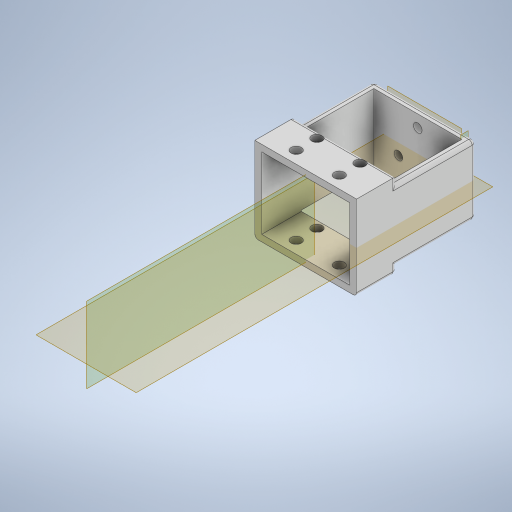
# Autodesk Inventor part: gripper-adapter
Saved by Autodesk Inventor 2024 (Build 280153000, 153)
## iProperties
Created: 2024-04-26
Part Number: gripper-adapter
Material: Generic
Document SubType Name: Modeling
Designer: MaartenGeorgesBuelen
Density: 1 g/cm^3
Appearance: Default
Author: MaartenGeorgesBuelen
## iProperties of the stored document gripper-adapter_3DPrint.ipt
Created: 2024-04-26
Part Number: gripper-adapter_3DPrint
Material: Generic
Document SubType Name: Modeling
Designer: MaartenGeorgesBuelen
Density: 1 g/cm^3
Appearance: Default
Author: MaartenGeorgesBuelen
Autodesk Inventor part; units mm, degrees
ref_plane "YZ Plane" through (0, 0, 0) normal (1, 0, 0) x (0, 1, 0)
ref_plane "XZ Plane" through (0, 0, 0) normal (0, 1, 0) x (-1, 0, 0)
ref_plane "Work Plane1" through (0, 0, 0) normal (0, 0, 1) x (1, 0, 0)
ref_plane "Work Plane7" through (25, -7, 170) normal (-1, 0, 0) x (0, 0, -1)
sketch "Sketch1" plane through (0, 0, 0) normal (0, 0, 1) x (1, 0, 0)
  circle A0 centre (0, 13) radius 5 projected
  line L0 (-15.25, 21.0877) -> (-12.5, 22.6754) projected
  line L1 (-12.5, 22.6754) -> (-9.75, 21.0877) projected
  line L2 (-9.75, 21.0877) -> (-9.75, 17.9123) projected
  line L3 (-9.75, 17.9123) -> (-12.5, 16.3246) projected
  line L4 (-12.5, 16.3246) -> (-15.25, 17.9123) projected
  line L5 (-15.25, 17.9123) -> (-15.25, 21.0877) projected
  line L6 (9.75, 21.0877) -> (12.5, 22.6754) projected
  line L7 (12.5, 22.6754) -> (15.25, 21.0877) projected
  line L8 (15.25, 21.0877) -> (15.25, 17.9123) projected
  line L9 (15.25, 17.9123) -> (12.5, 16.3246) projected
  line L10 (12.5, 16.3246) -> (9.75, 17.9123) projected
  line L11 (9.75, 17.9123) -> (9.75, 21.0877) projected
  circle A1 centre (-11.2583, 6.5) radius 1.5 projected
  circle A2 centre (11.2583, 6.5) radius 1.5 projected
  circle A3 centre (0, 26) radius 1.5 projected
  line L12 (-16.5, -4) -> (16.5, -4) projected
  line L13 (16.5, -4) -> (16.5, 0.0385) projected
  arc A4 (17.5169, 4.4322) -> (16.5, 0.0385) centre (26.5, 0.0385) ccw projected
  arc A5 (17.5169, 4.4322) -> (-17.5169, 4.4322) centre (0, 13) ccw projected
  arc A6 (-16.5, 0.0385) -> (-17.5169, 4.4322) centre (-26.5, 0.0385) ccw projected
  line L14 (-16.5, 0.0385) -> (-16.5, -4) projected
  line L15 (0, 39.8) -> (0, -11.3)
  line L16 (16.5, -7) -> (16.5, 33)
  line L17 (-5, -7) -> (-25, -7) projected
  line L18 (-25, 33) -> (-5, 33) projected
  line L19 (16.5, -7) -> (29.5, -7)
  line L20 (29.5, -7) -> (29.5, 33)
  line L21 (29.5, 33) -> (16.5, 33)
  line L22 (16.5, 33) -> (16.5, -7)
  line L23 (25, -21.52) -> (25, 50.02) projected
  line L24 (-16.5, -4) -> (-16.5, 0.0385)
  line L25 (-16.5, -7) -> (-16.5, 33)
  line L26 (-16.5, -7) -> (-29.5, -7)
  line L27 (-29.5, -7) -> (-29.5, 33)
  line L28 (-29.5, 33) -> (-16.5, 33)
  line L29 (-16.5, 33) -> (-16.5, -7)
  line L30 (16.5, -7) -> (-16.5, -7)
  line L31 (-16.5, 33) -> (16.7576, 33)
  circle A7 centre (11.2583, 6.5) radius 2.5
  circle A8 centre (-11.2583, 6.5) radius 2.5
  circle A9 centre (0, 26) radius 2.5
  point P0 (0, 0)
  point P1 (16.5, 23.3923)
  point P2 (-11.2583, 6.5)
  point P3 (-26.5, 0.0385)
  point P4 (25, -7)
  point P5 (25, 33)
  point P6 (-5, 33)
  dimension "d28" = 4.5
  dimension "d29" = 40
  dimension "d30" = 60
  dimension "d31" = 40
  dimension "d32" = 41.5
  dimension "d33" = 12.4413
  dimension "d34" = 8.5
  dimension "d35" = 4.1208
  dimension "d36" = 8.5
  dimension "d37" = 16.1041
  dimension "d38" = 8.5
  dimension "d39" = 16.1041
  dimension "d40" = 8.5
  dimension "d41" = 19.6016
  dimension "d60" = 1
  dimension "d61" = 1
  dimension "d62" = 1
  constraints: 28 end point, 7 symmetric about line, 3 centre point, 2 parallel, 1 collinear, 1 horizontal, 1 perpendicular, 1 point on line, 1 vertical, 2 other
  measures "d28" distance between parallel lines of L23 L20
  measures "d29" distance between parallel lines of L19 L21
  measures "d30" angle of L9 L25
  measures "d31" distance between parallel lines of L17 L21
  measures "d32" distance between parallel lines of L23 L29
  measures "d33" distance from line of L16.end L9
  measures "d34" distance from line of point (16.5, 23.392) L23
  measures "d35" distance from line of point (16.5, 23.392) L9
  measures "d36" distance from line of point (16.5, 0.039) L23
  measures "d37" distance from line of point (16.5, 0.039) L9
  measures "d38" distance from line of point (16.5, 0.039) L23
  measures "d39" distance from line of point (16.5, 0.039) L9
  measures "d40" distance from line of point (16.5, -4) L23
  measures "d41" distance from line of point (16.5, -4) L9
  measures "d60" radial gap between concentric circles of A2 A7
  measures "d61" radial gap between concentric circles of A1 A8
  measures "d62" radial gap between concentric circles of A3 A9
extrude "Extrusion1" add sketch "Sketch1" along normal blind 4 contours A0 L15 | A0 L15 A9 A5 L16 L13 L12 | L15 A0 | A0 L15 L12 L14 L25 A5 A9 | L15 L30 L17 L25 L12 | L12 L16 L30 L15 | L25 L17 L26 L27 L28 L18 A5 A6 L14 | L13 A4 A5 L16 L21 L23 L19 | L15 L31 L16 A5 | A5 L25 L18 L31 L15 | A6 A5 L25 | L16 A5 A4 | L23 L21 L20 L19 | L0 L1 L2 L3 L4 L5 | L6 L7 L8 L9 L10 L11
sketch "Sketch6" plane through (0, 0, 4) normal (0, 0, 1) x (1, 0, 0)
  line L0 (-29.5, 33) -> (-29.5, -7) projected
  line L1 (29.5, -7) -> (25.5, -7)
  line L2 (25.5, -7) -> (25.5, 33)
  line L3 (25.5, 33) -> (29.5, 33)
  line L4 (29.5, 33) -> (29.5, -7)
  line L5 (-29.5, -7) -> (-25.5, -7)
  line L6 (-25.5, -7) -> (-25.5, 33)
  line L7 (-25.5, 33) -> (-29.5, 33)
  line L8 (-29.5, 33) -> (-29.5, -7)
  line L9 (-29.5, -7) -> (29.5, -7) projected
  line L10 (29.5, -7) -> (29.5, 33) projected
  line L11 (29.5, 33) -> (-29.5, 33) projected
  point P0 (0, 0)
  dimension "d42" = 4
  dimension "d43" = 4
  dimension "d44" = 0
  dimension "d45" = 0
  constraints: 16 end point, 4 parallel, 2 horizontal, 2 perpendicular
  measures "d42" distance of L2.end L3.end
  measures "d43" distance of L7.end L6.end
  measures "d44" distance between parallel lines of L11 L3
  measures "d45" distance between parallel lines of L11 L7
extrude "Extrusion6" add sketch "Sketch6" along normal blind 65 contours L3 L4 L1 L2
sketch "Sketch7" plane through (-29.5, -7, 0) normal (0, -1, 0) x (1, 0, 0)
  line L0 (55, 69) -> (59, 69) projected
  line L1 (59, 0) -> (59, 69) projected
  line L2 (55, 69) -> (59, 69)
  line L3 (59, 69) -> (59, 46)
  line L4 (59, 46) -> (55, 46)
  line L5 (55, 46) -> (55, 69)
  point P0 (29.5, 0)
  dimension "d48" = 23
  constraints: 8 end point, 2 parallel, 1 horizontal, 1 perpendicular, 1 point on line
  measures "d48" distance of L2.end L3.end
extrude "Extrusion7" add sketch "Sketch7" along normal blind 4.5
sketch "Sketch8" plane through (25.5, -7, 4) normal (-1, 0, 0) x (0, 0, 1)
  line L0 (0, 0) -> (0, 40) projected
  line L1 (0, 0) -> (42, 0) projected
  line L2 (42, 0) -> (42, -4.5) projected
  line L3 (65, -4.5) -> (42, -4.5) projected
  line L4 (65, 40) -> (65, -4.5) projected
  line L5 (0, 40) -> (65, 40) projected
  line L6 (65, -4.5) -> (42, -4.5)
  line L7 (42, -4.5) -> (42, -0.7)
  line L8 (42, -0.7) -> (65, -0.7)
  line L9 (65, -0.7) -> (65, -4.5)
  point P0 (-4, 7)
  dimension "d51" = 3.8
  constraints: 8 end point, 2 parallel, 1 horizontal, 1 perpendicular, 1 point on line
  measures "d51" distance of L6.end L7.end
ref_plane "Work Plane8" through (0, -9, 64) normal (-1, 0, 0) x (0, 0, 1)
extrude "Extrusion8" add sketch "Sketch8" along normal up to surface (25.5 mm away) contours L8 L4 L3 L2
ref_plane "Work Plane9" through (0, 38, 140.8927) normal (-1, 0, 0) x (0, 1, 0)
ref_plane "Work Plane10" through (21, 13, 170) normal (0, 1, 0) x (1, 0, 0)
mirror "Mirror3" about plane through (0, 38, 140.8927) normal (-1, 0, 0) of "Extrusion6", "Extrusion7", "Extrusion8"
mirror "Mirror4" about plane through (21, 13, 170) normal (0, 1, 0) of "Extrusion6", "Extrusion7", "Extrusion8", "Mirror3"
sketch "Sketch9" plane through (-29.5, -11.5, 0) normal (0, -1, 0) x (1, 0, 0)
  circle A0 centre (17, 50) radius 1.95 projected
  circle A1 centre (42, 50) radius 1.95 projected
  circle A2 centre (17, 62) radius 1.95 projected
  circle A3 centre (42, 62) radius 1.95 projected
  line L0 (34.5, 30) -> (24.5, 30) projected
  arc A4 (34.5, 30) -> (54.5, 50) centre (34.5, 50) ccw projected
  line L1 (54.5, 150.4041) -> (54.5, 50) projected
  spline S0 degree 3 poles (58.5, 156.7335) (58.3042, 156.7335) (58.0717, 156.7001) (57.6735, 156.5882) (57.4345, 156.4826) (56.7488, 156.0807) (56.2679, 155.5825) (55.7145, 154.8068) (55.5061, 154.4513) (55.1512, 153.7098) (55.0043, 153.3239) (54.7718, 152.5757) (54.6684, 152.1401) (54.5324, 151.2582) (54.5, 150.8118) (54.5, 150.4041) knots 1.468489 1.468489 1.468489 1.468489 1.527225 1.527225 1.592556 1.592556 1.765662 1.765662 1.878422 1.878422 1.991181 1.991181 2.113494 2.113494 2.235806 2.235806 2.235806 2.235806 projected
  line L2 (58.5, 156.7335) -> (50.5, 156.7335) projected
  line L3 (50.5, 170) -> (50.5, 156.7335) projected
  line L4 (41.2, 170) -> (50.5, 170) projected
  line L5 (41.2, 170) -> (41.2, 122.921) projected
  line L6 (17.8, 122.921) -> (41.2, 122.921) projected
  line L7 (17.8, 170) -> (17.8, 122.921) projected
  line L8 (17.8, 170) -> (4.5, 170) projected
  line L9 (4.5, 170) -> (4.5, 50) projected
  arc A5 (4.5, 50) -> (24.5, 30) centre (24.5, 50) ccw projected
  circle A6 centre (42, 62) radius 2.95
  circle A7 centre (42, 50) radius 2.95
  circle A8 centre (17, 50) radius 2.95
  circle A9 centre (17, 62) radius 2.95
  point P0 (29.5, 0)
  dimension "d54" = 1
  dimension "d55" = 1
  dimension "d56" = 1
  dimension "d57" = 1
  constraints: 4 centre point
  measures "d54" radial gap between concentric circles of A3 A6
  measures "d55" radial gap between concentric circles of A1 A7
  measures "d56" radial gap between concentric circles of A0 A8
  measures "d57" radial gap between concentric circles of A2 A9
extrude "Extrusion9" cut sketch "Sketch9" against normal through all contours A0 | A1 | A2 | A3 | A6 | A7 | A8 | A9
fillet "Fillet4" radius 2 15 edges at (29.5, -11.5, 57.5) (29.5, -7, 23) (0, -7, 0) (-29.5, 13, 0) (-29.5, -7, 23) (-29.5, -11.5, 57.5) (-29.5, -9.25, 46) (29.5, -9.25, 46) (29.5, 35.25, 46) (29.5, 33, 23) (0, 37.5, 46) (0, -11.5, 46) (0, 33, 0) (-29.5, 33, 23) (29.5, 13, 0)
body "Solid1"
